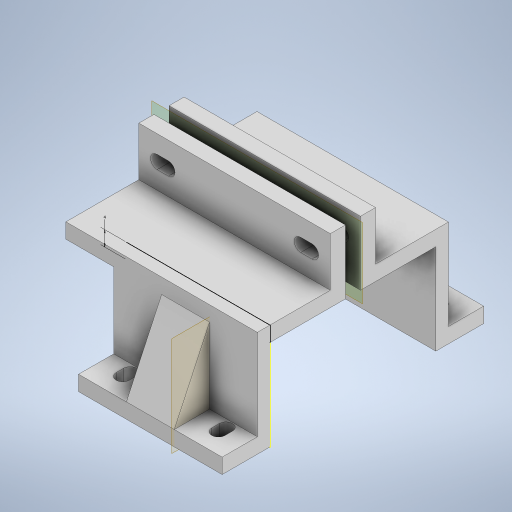
# Autodesk Inventor part: IRMountLeft
Saved by Autodesk Inventor 2023.1 (Build 271208000, 208)
## iProperties
Created: 2023-03-21
Part Number: IRMountLeft
Material: Generic
Document SubType Name: Modeling
Designer: bpat387
Density: 1 g/cm^3
Appearance: Default
Author: bpat387
## iProperties of the stored document IRMount_3DPrint.ipt
Created: 2023-03-23
Part Number: IRMount_3DPrint
Material: Generic
Document SubType Name: Modeling
Designer: bpat387
Density: 1 g/cm^3
Appearance: Default
Author: bpat387
Autodesk Inventor part; units mm, degrees
ref_plane "YZ Plane" through (0, 0, 0) normal (1, 0, 0) x (0, 1, 0)
ref_plane "XZ Plane" through (0, 0, 0) normal (0, 1, 0) x (-1, 0, 0)
ref_plane "XY Plane" through (0, 0, 0) normal (0, 0, 1) x (1, 0, 0)
sketch "Sketch1" plane through (0, 0, 0) normal (0, 1, 0) x (-1, 0, 0)
  line L0 (0, 0) -> (38.1, 0)
  line L1 (38.1, 0) -> (38.1, -12.7)
  line L2 (38.1, -12.7) -> (0, -12.7)
  line L3 (0, -12.7) -> (0, 0)
  line L4 (38.1, 0) -> (0, -12.7) construction
  line L5 (0, 0) -> (38.1, -12.7) construction
  line L6 (0, -6.35) -> (38.1, -6.35) construction
  line L7 (19.05, -6.35) -> (31.75, -6.35) construction
  line L8 (19.05, -6.35) -> (6.35, -6.35)
  line L9 (6.35, -5.35) -> (31.75, -5.35)
  line L10 (31.75, -5.35) -> (31.75, -7.35)
  line L11 (31.75, -7.35) -> (6.35, -7.35)
  line L12 (6.35, -7.35) -> (6.35, -5.35)
  line L13 (6.35, -5.35) -> (31.75, -7.35) construction
  line L14 (31.75, -5.35) -> (6.35, -7.35) construction
  circle A0 centre (31.75, -7.35) radius 1.75
  circle A1 centre (31.75, -5.35) radius 1.75
  line L15 (33.5, -5.35) -> (33.5, -7.35)
  line L16 (30, -7.35) -> (30, -5.35)
  circle A2 centre (6.35, -7.35) radius 1.75
  circle A3 centre (6.35, -5.35) radius 1.75
  line L17 (4.6, -7.35) -> (4.6, -5.35)
  line L18 (8.1, -7.35) -> (8.1, -5.35)
  dimension "d0" = 38.1
  dimension "d1" = 12.7
  dimension "d2" = 12.7
  dimension "d3" = 12.7
  dimension "d12" = 25.4
  dimension "d13" = 2
  dimension "d14" = 3.5
  dimension "d15" = 3.5
  dimension "d16" = 3.5
  dimension "d17" = 3.5
  constraints: 38 end point, 8 point on circle, 6 coincident, 6 tangent, 5 midpoint, 4 centre point, 4 parallel, 4 perpendicular, 3 point on line, 2 horizontal
  measures "d0" distance of L1.end L2.end
  measures "d1" distance of L2.end L0.start
  measures "d2" distance of L7.start L7.end
  measures "d3" distance of L7.start L8.end
  measures "d12" distance of L10.end L11.end
  measures "d13" distance between parallel lines of L9 L11
  measures "d14" diameter of A0
  measures "d15" diameter of A1
  measures "d16" diameter of A2
  measures "d17" diameter of A3
extrude "Extrusion1" add sketch "Sketch1" along normal blind 4 contours L0 L1 L2 L3 | L18 L9 L16 L11
sketch "Sketch2" plane through (0, 0, 0) normal (1, 0, 0) x (0, 0, -1)
  line L0 (0, 0) -> (12.7, 0) projected
  line L1 (12.7, 0) -> (12.7, 4) projected
  line L2 (0, 4) -> (12.7, 4) projected
  line L3 (0, 0) -> (0, 4) projected
  line L4 (12.7, 4) -> (9.35, 4)
  line L5 (9.35, 4) -> (9.35, 24)
  line L6 (9.35, 24) -> (12.7, 24)
  line L7 (12.7, 24) -> (12.7, 4)
  dimension "d8" = 24
  dimension "d9" = 3.35
  constraints: 8 end point, 2 parallel, 1 horizontal, 1 perpendicular
  measures "d8" distance between parallel lines of L0 L6
  measures "d9" distance between parallel lines of L5 L7
extrude "Extrusion2" add sketch "Sketch2" against normal up to surface (38.1 mm away) contours L2 L5 L6 L7
ref_plane "Work Plane1" through (-12.7, 0, 0) normal (1, 0, 0) x (0, 0, -1)
sketch "Sketch3" plane through (-12.7, 0, 0) normal (1, 0, 0) x (0, 0, -1)
  line L0 (0, 0) -> (12.7, 0) projected
  line L1 (12.7, 0) -> (12.7, 24) projected
  line L2 (12.7, 24) -> (9.35, 24) projected
  line L3 (9.35, 24) -> (9.35, 4) projected
  line L4 (0, 4) -> (9.35, 4) projected
  line L5 (0, 0) -> (0, 4) projected
  line L6 (0, 4) -> (9.35, 24)
  constraints: 2 end point
extrude "Extrusion3" add sketch "Sketch3" against normal blind 12.7 contours L6 L3 L4
sketch "Sketch4" plane through (0, 0, -12.7) normal (0, 0, -1) x (-1, 0, 0)
  line L0 (0, 0) -> (38.1, 0) projected
  line L1 (38.1, 0) -> (38.1, 24) projected
  line L2 (0, 24) -> (38.1, 24) projected
  line L3 (0, 0) -> (0, 24) projected
  line L4 (0, 24) -> (12.7, 24) projected
  line L5 (0, 24) -> (38.1, 24)
  line L6 (38.1, 24) -> (38.1, 28)
  line L7 (38.1, 28) -> (0, 28)
  line L8 (0, 28) -> (0, 24)
  point P0 (0, 0)
  dimension "d21" = 4
  constraints: 8 end point, 2 parallel, 1 horizontal, 1 perpendicular, 1 point on line
  measures "d21" distance of L6.end L5.end
extrude "Extrusion4" add sketch "Sketch4" against normal up to surface (3.35 mm away) contours L8 L7 L6 L2
extrude "Extrusion5" add sketch "Sketch4" along normal blind 20 contours L8 L7 L6 L2
sketch "Sketch5" plane through (-38.1, 0, -12.7) normal (-1, 0, 0) x (0, 0, 1)
  line L0 (0, 0) -> (12.7, 0) projected
  line L1 (12.7, 0) -> (12.7, 4) projected
  line L2 (3.35, 4) -> (12.7, 4) projected
  line L3 (3.35, 28) -> (3.35, 4) projected
  line L4 (-20, 28) -> (3.35, 28) projected
  line L5 (-20, 24) -> (-20, 28) projected
  line L6 (0, 24) -> (-20, 24) projected
  line L7 (0, 0) -> (0, 24) projected
  line L8 (-20, 24) -> (-20, 28) projected
  line L9 (3.35, 28) -> (3.35, 4) projected
  line L10 (-20, 24) -> (3.35, 24)
  line L11 (3.35, 24) -> (3.35, 28)
  line L12 (3.35, 28) -> (-20, 28)
  line L13 (-20, 28) -> (-20, 24)
  point P0 (12.7, 0)
  constraints: 8 end point, 2 parallel, 1 horizontal, 1 perpendicular
extrude "Extrusion6" add sketch "Sketch5" along normal blind 12.7 contours L6 L5 L4 L3 L10
sketch "Sketch6" plane through (0, 28, -9.35) normal (0, 1, 0) x (1, 0, 0)
  line L0 (0, 0) -> (0, 23.35) projected
  line L1 (0, 23.35) -> (-50.8, 23.35)
  line L2 (-50.8, 23.35) -> (-50.8, 19.35)
  line L3 (-50.8, 19.35) -> (0, 19.35)
  line L4 (0, 19.35) -> (0, 23.35)
  point P0 (0, -9.35)
  point P1 (0, 19.35)
  dimension "d28" = 4
  constraints: 8 end point, 2 parallel, 1 horizontal, 1 perpendicular
  measures "d28" distance between parallel lines of L1 L3
extrude "Extrusion7" add sketch "Sketch6" along normal blind 13
sketch "Sketch7" plane through (-50.8, 28, -28.7) normal (0, 0, 1) x (1, 0, 0)
  line L0 (50.8, 0) -> (0, 0) projected
  line L1 (50.8, 0) -> (50.8, 13) projected
  line L2 (0, 13) -> (50.8, 13) projected
  line L3 (0, 0) -> (0, 13) projected
  line L4 (0, -4) -> (0, 13) projected
  line L5 (0, 13) -> (6.35, 13)
  line L6 (6.35, 13) -> (6.35, 0) construction
  line L7 (6.35, 0) -> (0, 0)
  line L8 (0, 0) -> (0, 13)
  line L9 (50.8, 0) -> (0, 0) projected
  line L10 (50.8, -4) -> (50.8, 13) projected
  line L11 (50.8, 13) -> (44.45, 13)
  line L12 (44.45, 13) -> (44.45, 0) construction
  line L13 (44.45, 0) -> (50.8, 0)
  line L14 (50.8, 0) -> (50.8, 13)
  line L15 (6.35, 6.5) -> (44.45, 6.5) construction
  line L16 (42.95, 7.5) -> (45.95, 7.5) construction
  line L17 (45.95, 7.5) -> (45.95, 5.5) construction
  line L18 (45.95, 5.5) -> (42.95, 5.5) construction
  line L19 (42.95, 5.5) -> (42.95, 7.5) construction
  line L20 (42.95, 7.5) -> (45.95, 5.5) construction
  line L21 (45.95, 7.5) -> (42.95, 5.5) construction
  line L22 (4.85, 5.5) -> (7.85, 5.5) construction
  line L23 (7.85, 5.5) -> (7.85, 7.5) construction
  line L24 (7.85, 7.5) -> (4.85, 7.5) construction
  line L25 (4.85, 7.5) -> (4.85, 5.5) construction
  line L26 (4.85, 5.5) -> (7.85, 7.5) construction
  line L27 (7.85, 5.5) -> (4.85, 7.5) construction
  line L28 (4.85, 6.5) -> (7.85, 6.5) construction
  line L29 (4.85, 4.75) -> (7.85, 4.75)
  line L30 (7.85, 8.25) -> (4.85, 8.25)
  arc A0 (4.85, 8.25) -> (4.85, 4.75) centre (4.85, 6.5) ccw
  arc A1 (7.85, 4.75) -> (7.85, 8.25) centre (7.85, 6.5) ccw
  line L31 (42.95, 6.5) -> (45.95, 6.5) construction
  line L32 (42.95, 4.75) -> (45.95, 4.75)
  line L33 (45.95, 8.25) -> (42.95, 8.25)
  arc A2 (42.95, 8.25) -> (42.95, 4.75) centre (42.95, 6.5) ccw
  arc A3 (45.95, 4.75) -> (45.95, 8.25) centre (45.95, 6.5) ccw
  point P0 (50.8, -28)
  dimension "d31" = 6.35
  dimension "d32" = 6.35
  dimension "d33" = 3
  dimension "d34" = 2
  dimension "d35" = 3
  dimension "d36" = 2
  dimension "d37" = 3.5
  dimension "d38" = 3.5
  constraints: 58 end point, 12 midpoint, 10 parallel, 8 point on circle, 8 tangent, 4 centre point, 4 horizontal, 4 perpendicular, 2 point on line
  measures "d31" distance between parallel lines of L3 L6
  measures "d32" distance between parallel lines of L1 L12
  measures "d33" distance of L17.end L18.end
  measures "d34" distance of L16.end L17.end
  measures "d35" distance of L24.end L23.end
  measures "d36" distance of L23.end L22.end
  measures "d37" diameter of A1
  measures "d38" diameter of A3
extrude "Extrusion8" cut sketch "Sketch7" against normal up to surface (4 mm away) contours A0 L30 A1 L29 | A2 L33 A3 L32
ref_plane "Work Plane2" through (0, 0, -34.7) normal (0, 0, -1) x (-1, 0, 0)
mirror "Mirror1" about plane through (0, 0, -34.7) normal (0, 0, -1)
